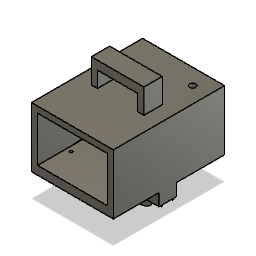
Enclosure v9 (Autodesk Fusion 360 design; units mm, degrees)
Autodesk Fusion 360 part; units mm, degrees
note: some values were not read from the file. Set by a fixed rule: which sketch regions a step uses.
sketch "Sketch1" plane through (0, 0, 0) normal (0, 0, 1) x (1, 0, 0)
  line L0 (0, 0) -> (67, 0)
  line L1 (67, 0) -> (67, 47)
  line L2 (67, 47) -> (0, 47)
  line L3 (0, 47) -> (0, 0)
  dimension "d1" = 47
  dimension "d2" = 67
  constraint horizontal L0
  constraint vertical L1
  constraint horizontal L2
  constraint vertical L3
  constraint coincident L0.start L3.end
  measures "d1" distance of L0.start L2.end
  measures "d2" distance of L0.start L0.end
extrude "Extrude1" add sketch "Sketch1" against normal blind 91 makes body 1
shell "Shell1" thickness 5 removed faces 1 at (22.3333, 15.6667, 0) on bodies 1
sketch "Sketch2" plane through (0, 42, 0) normal (0, -1, 0) x (1, 0, 0)
  line L0 (5, -86) -> (62, -86)
  line L1 (62, 0) -> (5, 0)
  circle A0 centre (9, -17) radius 1.2
  circle A1 centre (58, -17) radius 1.2
  circle A2 centre (42, -67.5) radius 1.2
  circle A3 centre (14, -67.5) radius 1.2
  circle A4 centre (54, -78) radius 2.5
  line L2 (62, -86) -> (62, 0)
  line L3 (5, 0) -> (5, -86)
  dimension "d16" = 2.4
  dimension "d17" = 17
  dimension "d18" = 2.4
  dimension "d19" = 17
  dimension "d20" = 49
  dimension "d23" = 2.4
  dimension "d24" = 50.5
  dimension "d26" = 2.4
  dimension "d27" = 28
  dimension "d28" = 50.5
  dimension "d41" = 5
  dimension "d48" = 5
  dimension "d49" = 8
  measures "d16" diameter of A0
  measures "d17" distance of L1 A0.centre
  measures "d18" diameter of A1
  measures "d19" distance of L1 A1.centre
  measures "d20" distance of A0.centre A1.centre
  measures "d23" diameter of A2
  measures "d24" vertical distance of A1.centre A2.centre
  measures "d26" diameter of A3
  measures "d27" horizontal distance of A2.centre A3.centre
  measures "d28" vertical distance of A0.centre A3.centre
  measures "d41" horizontal distance of A0.centre A3.centre
  measures "d48" diameter of A4
  measures "d49" distance of L0 A4.centre
hole "Hole1" at (9, 42, -17) direction (0, 1, 0) diameter 2.4 depth 4 tip angle 180 bodies 1
hole "Hole2" at (58, 42, -17) direction (0, 1, 0) diameter 2.4 depth 4 tip angle 180 bodies 1
hole "Hole5" at (14, 42, -67.5) direction (0, 1, 0) diameter 2.4 depth 4 tip angle 180 bodies 1
hole "Hole6" at (42, 42, -67.5) direction (0, 1, 0) diameter 2.4 depth 4 tip angle 180 bodies 1
hole "Hole7" at (54, 42, -78) direction (0, 1, 0) diameter 5 end through all bodies 1
sketch "Sketch3" plane through (0, 5, 0) normal (0, 1, 0) x (-1, 0, 0)
  line L0 (-5, 0) -> (-62, 0)
  line L1 (-62, -86) -> (-5, -86)
  circle A0 centre (-9, -23.5) radius 1.2
  circle A1 centre (-58, -23.5) radius 1.2
  circle A2 centre (-9, -81.5) radius 1.2
  circle A3 centre (-58, -81.5) radius 1.2
  line L2 (-62, 0) -> (-62, -86)
  line L3 (-5, -86) -> (-5, 0)
  dimension "d54" = 2.4
  dimension "d55" = 23.5
  dimension "d56" = 2.4
  dimension "d57" = 23.5
  dimension "d58" = 49
  dimension "d60" = 2.4
  dimension "d61" = 58
  dimension "d63" = 2.4
  dimension "d64" = 49
  dimension "d65" = 58
  measures "d54" diameter of A0
  measures "d55" distance of L0 A0.centre
  measures "d56" diameter of A1
  measures "d57" distance of L0 A1.centre
  measures "d58" distance of A0.centre A1.centre
  measures "d60" diameter of A2
  measures "d61" vertical distance of A0.centre A2.centre
  measures "d63" diameter of A3
  measures "d64" horizontal distance of A2.centre A3.centre
  measures "d65" distance of A1.centre A3.centre
sketch "Sketch4" plane through (0, 0, 0) normal (-1, 0, 0) x (0, 0, 1)
  line L0 (0, 0) -> (0, 47)
  line L1 (0, 47) -> (-91, 47)
  line L2 (-91, 47) -> (-91, 0)
  line L3 (-91, 0) -> (0, 0)
  line L4 (-81, 2.1) -> (-30, 2.1)
  line L5 (-30, 2.1) -> (-30, 5.4)
  line L6 (-30, 5.4) -> (-81, 5.4)
  line L7 (-81, 5.4) -> (-81, 2.1)
  dimension "d78" = 10
  dimension "d79" = 2.1
  dimension "d80" = 3.3
  dimension "d81" = 51
  constraint horizontal L4
  constraint vertical L5
  constraint horizontal L6
  constraint vertical L7
  measures "d78" distance of L2 L7
  measures "d79" distance of L3 L4
  measures "d80" distance of L4.start L6.end
  measures "d81" distance of L5.end L6.end
extrude "Extrude5" cut sketch "Sketch4" against normal blind 5 contours L4 L5 L6 L7 bodies 1
extrude "Extrude6" add 1 faces at (22.3333, 0, -30.3333) along direction (0, -1, 0) blind 12 on bodies 1 bodies 1
hole "Hole12" at (9, 5, -81.5) direction (0, -1, 0) diameter 2.4 depth 4 tip angle 180 bodies 1
hole "Hole13" at (58, 5, -81.5) direction (0, -1, 0) diameter 2.4 depth 4 tip angle 180 bodies 1
hole "Hole14" at (9, 5, -23.5) direction (0, -1, 0) diameter 2.4 depth 4 tip angle 180 bodies 1
hole "Hole15" at (58, 5, -23.5) direction (0, -1, 0) diameter 2.4 depth 4 tip angle 180 bodies 1
sketch "Sketch9" plane through (0, -12, 0) normal (0, -1, 0) x (1, 0, 0)
  line L0 (67, 0) -> (0, 0)
  line L1 (0, 0) -> (0, -91)
  line L2 (0, -91) -> (67, -91)
  line L3 (67, -91) -> (67, 0)
  line L4 (6, -40.35) -> (31, -40.35)
  line L5 (31, -40.35) -> (31, -48.55)
  line L6 (31, -48.55) -> (6, -48.55)
  line L7 (6, -48.55) -> (6, -40.35)
  line L8 (36, -40.35) -> (61, -40.35)
  line L9 (61, -40.35) -> (61, -48.55)
  line L10 (61, -48.55) -> (36, -48.55)
  line L11 (36, -48.55) -> (36, -40.35)
  line L12 (6, -40.35) -> (28.5, -40.35)
  line L13 (6, -48.55) -> (28.4996, -48.55)
  line L14 (36, -40.35) -> (61, -40.35)
  line L15 (36, -48.55) -> (61, -48.55)
  line L16 (6, -40.35) -> (67, -40.35)
  line L17 (67, -40.35) -> (67, -39.35)
  line L18 (67, -39.35) -> (6, -39.35)
  line L19 (6, -39.35) -> (6, -40.35)
  line L20 (6, -48.55) -> (67, -48.55)
  line L21 (67, -48.55) -> (67, -49.55)
  line L22 (67, -49.55) -> (6, -49.55)
  line L23 (6, -49.55) -> (6, -48.55)
  line L24 (6, -48.55) -> (0, -48.55)
  line L25 (0, -48.55) -> (0, -49.55)
  line L26 (0, -49.55) -> (6, -49.55)
  line L27 (6, -49.55) -> (6, -48.55)
  line L28 (6, -40.35) -> (0, -40.35)
  line L29 (0, -40.35) -> (0, -39.35)
  line L30 (0, -39.35) -> (6, -39.35)
  line L31 (6, -39.35) -> (6, -40.35)
  dimension "d100" = 8.2
  dimension "d101" = 25
  dimension "d102" = 40.35
  dimension "d103" = 8.2
  dimension "d104" = 25
  dimension "d105" = 40.35
  dimension "d106" = 6
  dimension "d107" = 6
  dimension "d116" = 1
  dimension "d117" = 1
  dimension "d119" = 1
  dimension "d120" = 1
  constraint horizontal L4
  constraint vertical L5
  constraint horizontal L6
  constraint vertical L7
  constraint horizontal L8
  constraint vertical L9
  constraint horizontal L10
  constraint vertical L11
  constraint horizontal L12
  constraint horizontal L13
  constraint horizontal L14
  constraint horizontal L15
  constraint horizontal L16
  constraint vertical L17
  constraint horizontal L18
  constraint vertical L19
  constraint horizontal L20
  constraint vertical L21
  constraint horizontal L22
  constraint vertical L23
  constraint horizontal L24
  constraint vertical L25
  constraint horizontal L26
  constraint vertical L27
  constraint horizontal L28
  constraint vertical L29
  constraint horizontal L30
  constraint vertical L31
  constraint coincident L1 L29.end
  constraint collinear L3 L17
  constraint collinear L3 L21
  measures "d100" distance of L4.start L6.end
  measures "d101" distance of L4.start L4.end
  measures "d102" distance of L0 L4
  measures "d103" distance of L8.start L10.end
  measures "d104" distance of L8.end L8.start
  measures "d105" vertical distance of L0.start L8.end
  measures "d106" distance of L3 L9
  measures "d107" distance of L1 L7
  measures "d116" distance of L4.start L18.end
  measures "d117" distance of L6.end L22.end
  measures "d119" distance of L6.end L22.end
  measures "d120" distance of L4.start L18.end
extrude "Extrude7" cut sketch "Sketch9" against normal blind 15.2 contours L8 L9 L10 L11 L14 L15 L16 L20 | L4 L5 L6 L7 L12 L13 L16 L20 bodies 1
extrude "Extrude9" add sketch "Sketch9" along normal blind 1 contours L3 L4 L8 L12 L14 L16 L17 L18 L19 L31 | L1 L19 L28 L29 L30 L31 | L3 L6 L10 L13 L15 L20 L21 L22 L23 L27 | L1 L23 L24 L25 L26 L27 bodies 1
extrude "Extrude12" cut 1 faces at (22.3333, -12, -63.3667) along direction (0, 1, 0) blind 10 on bodies 1 bodies 1
extrude "Extrude13" cut 1 faces at (22.3333, -12, -13.1167) along direction (0, 1, 0) blind 10 on bodies 1 bodies 1
sketch "Sketch10" plane through (0, 0, -49.55) normal (0, 0, -1) x (-1, 0, 0)
  line L0 (-67, -2) -> (-67, -13)
  line L1 (-67, -13) -> (0, -13)
  line L2 (0, -13) -> (0, -2)
  line L3 (-67, -12) -> (0, -12)
  line L4 (0, -2) -> (-67, -2)
  dimension "d135" = 1
  constraint coincident L0 L3.start
  constraint coincident L2 L3.end
  constraint perpendicular L2 L3
  measures "d135" distance of L1 L3
sketch "Sketch11" plane through (0, 0, -39.35) normal (0, 0, 1) x (1, 0, 0)
  line L0 (0, -2) -> (0, -13)
  line L1 (0, -13) -> (67, -13)
  line L2 (67, -13) -> (67, -2)
  line L3 (0, -12) -> (67, -12)
  line L4 (67, -2) -> (0, -2)
  dimension "d136" = 1
  constraint coincident L0 L3.start
  constraint coincident L2 L3.end
  constraint perpendicular L2 L3
  measures "d136" distance of L1 L3
extrude "Extrude16" add sketch "Sketch10" along normal blind 2 contours L0 L2 L3 L4 bodies 1
extrude "Extrude17" add sketch "Sketch11" along normal blind 2 contours L0 L2 L3 L4 bodies 1
sketch "Sketch12" plane through (0, 0, -51.55) normal (0, 0, -1) x (-1, 0, 0)
  line L0 (-67, -12) -> (0, -12)
  line L1 (0, -12) -> (0, -2)
  line L2 (-67, -2) -> (-67, -12)
  circle A0 centre (-48.5, -9) radius 1
  circle A1 centre (-18.5, -9) radius 1
  line L3 (0, -2) -> (-67, -2)
  dimension "d141" = 2
  dimension "d142" = 3
  dimension "d143" = 18.5
  dimension "d144" = 2
  dimension "d145" = 3
  dimension "d146" = 18.5
  measures "d141" diameter of A0
  measures "d142" distance of L0 A0.centre
  measures "d143" distance of L2 A0.centre
  measures "d144" diameter of A1
  measures "d145" distance of L0 A1.centre
  measures "d146" distance of L1 A1.centre
hole "Hole16" at (18.5, -9, -51.55) direction (0, 0, 1) diameter 2 end through all bodies 1
hole "Hole17" at (48.5, -9, -51.55) direction (0, 0, 1) diameter 2 end through all bodies 1
copy_body "Body->Comp1" bodies 1 removing the originals makes body 2 in component "Boksen"
cylinder "CylinderPrimitive1" add diameter 2 height 14.2 placed x (1, 0, 0) y (0, 1, 0) z (0, 0, 1) at (10, -10, 0) separate body makes body 3 in component "Akslinger"
copy_body "CopyPasteBodies1" bodies 3 makes body 4 in component "Akslinger"
move_body "Move1" bodies 4 to x (1, 0, 0) y (0, 1, 0) z (0, 0, 1) at (30, 0, 0) in component "Akslinger"
cylinder "CylinderPrimitive3" add diameter 24 height 7.8 placed x (1, 0, 0) y (0, 1, 0) z (0, 0, 1) at (125, 0, 0) separate body makes body 5 in component "Hjul"
sketch "Sketch10 (2)" plane through (0, 0, 0) normal (0, 0, -1) x (-1, 0, 0) in component "Hjul"
  circle A0 centre (-125, 0) radius 12
  circle A1 centre (-125, 0) radius 1
  dimension "d194" = 2
  constraint concentric A0 A1
  measures "d194" diameter of A1
hole "Hole3" at (125, 0, 0) direction (0, 0, 1) diameter 2 end through all bodies 5 in component "Hjul"
copy_body "CopyPasteBodies1'" bodies 5 makes body 6 in component "Hjul"
move_body "Move1'" bodies 6 to x (1, 0, 0) y (0, 1, 0) z (0, 0, 1) at (30, 0, 0) in component "Hjul"
sketch "Sketch1 (2)" plane through (0, 47, 0) normal (0, 1, 0) x (-1, 0, 0) in component "Kamerastand"
  circle A0 centre (-54, -78) radius 2.5
  line L0 (0, 0) -> (-67, 0)
  line L1 (-67, 0) -> (-67, -91)
  line L2 (-67, -91) -> (0, -91)
  line L3 (0, -91) -> (0, 0)
  line L4 (-12, -52) -> (-17, -52)
  line L5 (-17, -52) -> (-17, -37)
  line L6 (-17, -37) -> (-12, -37)
  line L7 (-12, -37) -> (-12, -52)
  line L8 (-50, -52) -> (-55, -52)
  line L9 (-55, -52) -> (-55, -37)
  line L10 (-55, -37) -> (-50, -37)
  line L11 (-50, -37) -> (-50, -52)
  dimension "d202" = 15
  dimension "d203" = 15
  dimension "d204" = 37
  dimension "d205" = 37
  dimension "d206" = 12
  dimension "d207" = 12
  constraint horizontal L4
  constraint vertical L5
  constraint horizontal L6
  constraint vertical L7
  constraint horizontal L8
  constraint vertical L9
  constraint horizontal L10
  constraint vertical L11
  measures "d202" distance of L4.start L6.end
  measures "d203" distance of L8.start L10.end
  measures "d204" distance of L0 L6
  measures "d205" distance of L0 L10
  measures "d206" distance of L1 L9
  measures "d207" distance of L3 L7
extrude "Extrude1'" add sketch "Sketch1 (2)" along normal blind 20 separate body contours L4 L5 L6 L7 | L8 L9 L10 L11 makes body 7 at (17, 53.6667, -47) makes body 8 at (55, 53.6667, -47) in component "Kamerastand"
sketch "Sketch2 (2)" plane through (50, 0, 0) normal (-1, 0, 0) x (0, 0, 1) in component "Kamerastand"
  line L0 (-52, 47) -> (-37, 47)
  line L1 (-37, 47) -> (-37, 67)
  line L2 (-37, 67) -> (-52, 67)
  line L3 (-52, 67) -> (-52, 47)
  line L4 (-52, 67) -> (-37, 67)
  line L5 (-37, 67) -> (-37, 60)
  line L6 (-37, 60) -> (-52, 60)
  line L7 (-52, 60) -> (-52, 67)
  dimension "d210" = 7
  constraint horizontal L4
  constraint vertical L5
  constraint horizontal L6
  constraint vertical L7
  constraint coincident L2.end L3.start
  measures "d210" distance of L2.end L6.end
extrude "Extrude2" add sketch "Sketch2 (2)" along normal blind 33 contours L1 L2 L3 L4 L5 L6 L7 bodies 7 8 in component "Kamerastand"
component "Akslinger" placed x (1, 0, 0) y (0, 1, 0) z (0, 0, 1) at (8.5, 1, -51.55)
component "Boksen" placed x (1, 0, 0) y (0, 1, 0) z (0, 0, 1) at (0, 0, 0)
component "Hjul" placed x (1, 0, 0) y (0, 1, 0) z (0, 0, 1) at (-106.5, -9, -48.35)
component "Kamerastand" placed x (1, 0, 0) y (0, 1, 0) z (0, 0, 1) at (0, 0, 0)
named bodies: "Boks", "Aksling1", "Aksling2"
